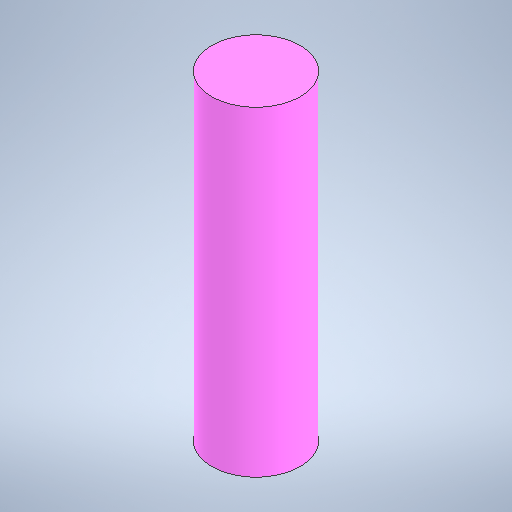
# Autodesk Inventor part: cellsplaceholder
Saved by Autodesk Inventor 2025.2 (Build 292293000, 293)
## iProperties
Created: 2024-11-26
Part Number: cellsplaceholder
Material: Generic
Document SubType Name: Modeling
Designer: cbast
Density: 1 g/cm^3
Appearance: Default
Author: cbast
Autodesk Inventor part; units mm, degrees
ref_plane "YZ Plane" through (0, 0, 0) normal (1, 0, 0) x (0, 1, 0)
ref_plane "XZ Plane" through (0, 0, 0) normal (0, 1, 0) x (-1, 0, 0)
ref_plane "XY Plane" through (0, 0, 0) normal (0, 0, 1) x (1, 0, 0)
sketch "Sketch1" plane through (0, 0, 0) normal (0, 1, 0) x (-1, 0, 0)
  circle A0 centre (0, 0) radius 9
  line L0 (0, 0) -> (0, -61.3231) construction
  line L1 (0, 0) -> (-21.4722, 0) construction
  line L2 (0, -61.3231) -> (0, -76.3064) construction
  dimension "d0" = 18
  constraints: 6 end point, 2 vertical, 1 centre point, 1 coincident, 1 horizontal
  measures "d0" diameter of A0
extrude "Extrusion1" add sketch "Sketch1" along normal blind 65
body "Solid1"
